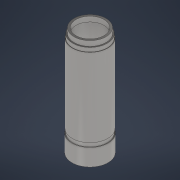
# Autodesk Inventor part: TestPiece1
Saved by Autodesk Inventor 2022 (Build 260153000, 153)
## iProperties
Created: 2024-05-07
Part Number: TestPiece1
Material: Generic
Document SubType Name: Modeling
Designer: jo_ki
Density: 1 g/cm^3
Appearance: Steel - Polished
Author: jo_ki
Autodesk Inventor part; units mm, degrees
ref_plane "YZ Plane" through (0, 0, 0) normal (1, 0, 0) x (0, 1, 0)
ref_plane "XZ Plane" through (0, 0, 0) normal (0, 1, 0) x (-1, 0, 0)
ref_plane "XY Plane" through (0, 0, 0) normal (0, 0, 1) x (1, 0, 0)
sketch "Sketch3" plane through (0, 0, 0) normal (0, 0, 1) x (1, 0, 0)
  line L0 (0, 0) -> (18.25, 0)
  line L1 (18.25, 0) -> (18.25, 86.5)
  line L2 (18.25, 86.5) -> (0, 86.5)
  line L3 (0, 86.5) -> (0, 0)
  line L4 (18.25, 4) -> (18.75, 4)
  line L5 (18.75, 4) -> (18.75, 82.5)
  line L6 (18.75, 82.5) -> (18.25, 82.5)
  line L7 (18.25, 82.5) -> (18.25, 4)
  line L8 (0, -94.8) -> (0, 204.8) projected
  line L9 (22, -29.5) -> (22, -33.5)
  line L10 (22, -33.5) -> (19, -52)
  line L11 (19, -52) -> (0, -52)
  line L12 (0, -52) -> (0, 0)
  line L13 (18.25, 0) -> (20.5, -17)
  line L14 (20.5, -17) -> (20.5, -23.5)
  line L15 (20.5, -23.5) -> (22, -29.5)
  line L16 (16, -52) -> (16, 106.5)
  line L17 (-4.4, 0) -> (26.4, 0) construction
  line L18 (18.25, 86.5) -> (20.5, 86.5)
  line L19 (20.5, 86.5) -> (22, 109.5)
  line L20 (22, 109.5) -> (22, 110.5)
  line L21 (22, 110.5) -> (21.5, 110.5)
  line L22 (21.5, 110.5) -> (21.5, 112)
  line L23 (21.5, 112) -> (22, 112)
  line L24 (22, 112) -> (22, 123)
  line L25 (22, 123) -> (21.5, 123.5)
  line L26 (21.5, 123.5) -> (21.5, 132.5)
  line L27 (21.5, 132.5) -> (22, 133)
  line L28 (22, 133) -> (22, 144)
  line L29 (22, 144) -> (21.5, 144)
  line L30 (21.5, 144) -> (21.5, 145.5)
  line L31 (21.5, 145.5) -> (22, 145.5)
  line L32 (22, 145.5) -> (22, 146.5)
  line L33 (22, 146.5) -> (19, 158.5)
  line L34 (19, 158.5) -> (19, 162)
  line L35 (19, 162) -> (0, 162)
  line L36 (16, 106.5) -> (16, 162)
  line L37 (14, 162) -> (14, 152)
  line L38 (14, 152) -> (16, 152)
  line L39 (18, 0) -> (18, -17)
  line L40 (18, -17) -> (20.5, -17)
  line L41 (20.5, 86.5) -> (15.25, 86.5)
  line L42 (15.25, 86.5) -> (15.25, 88.5)
  line L43 (15.25, 88.5) -> (20.5, 88.5)
  line L44 (20.5, 88.5) -> (20.5, 86.5)
  line L45 (15.25, 88.5) -> (17.25, 88.5)
  line L46 (17.25, 88.5) -> (17.25, 82.5)
  line L47 (17.25, 82.5) -> (15.25, 82.5)
  line L48 (15.25, 82.5) -> (15.25, 88.5)
  line L49 (15.25, 82.5) -> (17.75, 82.5)
  line L50 (17.75, 82.5) -> (17.75, 4)
  line L51 (17.75, 4) -> (15.25, 4)
  line L52 (15.25, 4) -> (15.25, 82.5)
  line L53 (15.25, 4) -> (17.25, 4)
  line L54 (17.25, 4) -> (17.25, 0)
  line L55 (17.25, 0) -> (15.25, 0)
  line L56 (15.25, 0) -> (15.25, 4)
  line L57 (15.25, 0) -> (18.25, 0)
  line L58 (18.25, 0) -> (18.25, -2)
  line L59 (18.25, -2) -> (15.25, -2)
  line L60 (15.25, -2) -> (15.25, 0)
  line L61 (18, -17) -> (16, -17)
  line L62 (16, 86.5) -> (14, 86.5)
  line L63 (14, 86.5) -> (14, 91.5)
  line L64 (14, 91.5) -> (16, 91.5)
  line L65 (16, 91.5) -> (16, 86.5)
  point P0 (18.25, 82.5)
  point P1 (16, 0)
  point P2 (16, 86.5)
  point P3 (20.4357, -17)
  point P4 (16, 0)
  point P5 (17.25, 4)
  point P6 (17.25, 86.5)
  point P7 (16, 108.5)
  point P8 (16, -2)
  point P9 (17.25, 0)
  point P10 (15.25, 86.5)
  point P11 (16, 88.5)
  point P12 (14, 88.5)
  dimension "d3" = 86.5
  dimension "d4" = 36.5
  dimension "d5" = 0.5
  dimension "d6" = 4
  dimension "d7" = 4
  dimension "d29" = 41
  dimension "d30" = 44
  dimension "d32" = 23.5
  dimension "d33" = 29.5
  dimension "d34" = 33.5
  dimension "d35" = 52
  dimension "d36" = 38
  dimension "d42" = 41
  dimension "d43" = 44
  dimension "d44" = 109.5
  dimension "d45" = 110.5
  dimension "d46" = 43
  dimension "d47" = 112
  dimension "d48" = 123
  dimension "d49" = 45
  dimension "d50" = 43
  dimension "d51" = 133
  dimension "d52" = 158.5
  dimension "d53" = 38
  dimension "d54" = 162
  dimension "d60" = 10
  dimension "d61" = 28
  dimension "d81" = 17
  dimension "d83" = 36
  dimension "d97" = 32
  dimension "d98" = 2
  dimension "d99" = 2
  dimension "d100" = 0.5
  dimension "d102" = 2
  dimension "d103" = 2
  dimension "d104" = 5
  dimension "d105" = 37.5
  dimension "d106" = 35.5
  constraints: 128 end point, 24 perpendicular, 18 parallel, 18 point on line, 9 horizontal, 5 equal length, 4 collinear, 2 vertical
  measures "d3" distance between parallel lines of L0 L2
  measures "d4" diameter of L1 L8
  measures "d5" distance between parallel lines of L1 L5
  measures "d6" distance from line of L1.end L6
  measures "d7" distance between parallel lines of L0 L4
  measures "d29" diameter of L13.end L8
  measures "d30" diameter of L9.start L8
  measures "d32" distance from line of L17 L14.end
  measures "d33" distance from line of L9.start L17
  measures "d34" distance from line of L17 L9.end
  measures "d35" distance from line of L17 L10.end
  measures "d36" diameter of L10.end L8
  measures "d42" diameter of L18.end L8
  measures "d43" diameter of L19.end L8
  measures "d44" distance from line of L17 L19.end
  measures "d45" distance from line of L17 L20.end
  measures "d46" diameter of L21.end L8
  measures "d47" distance from line of L17 L23.end
  measures "d48" distance from line of L17 L24.end
  measures "d49" angle of L24 L25
  measures "d50" diameter of L26 L8
  measures "d51" distance from line of L17 L27.end
  measures "d52" distance from line of L17 L33.end
  measures "d53" diameter of L33.end L8
  measures "d54" distance from line of L17 L34.end
  measures "d60" distance of L37.start L37.end
  measures "d61" diameter of L37 L8
  measures "d81" distance between parallel lines of L40 L0
  measures "d83" diameter of L39 L8
  measures "d97" diameter of L36 L8
  measures "d98" distance between parallel lines of L43 L2
  measures "d99" distance between parallel lines of L42 L46
  measures "d100" distance between parallel lines of L46 L50
  measures "d102" distance between parallel lines of L59 L0
  measures "d103" distance between parallel lines of L16 L63
  measures "d104" distance between parallel lines of L62 L64
  measures "d105" diameter of L5 L8
  measures "d106" diameter of L50 L8
revolve "Revolution1" add sketch "Sketch3" angle 360 about axis through (0, -10, 0) along (0, 1, 0) contours L56 L51 L16 L0 | L0 L16 L59 L60 | L16 L51 L54 L0 | L0 L39 L59 L16 | L52 L47 L16 L51 | L63 L64 L16 L43 L42 L2 | L59 L39 L61 L16 | L16 L47 L49 L50 L51 | L48 L2 L16 L47 | L42 L43 L16 L2 | L16 L2 L46 L47
equation "\"d7\" = d6"
equation "\"d50\" = d46"
body "Solid2"
